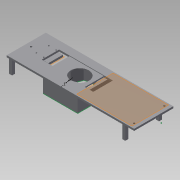
# Autodesk Inventor part: 10_Grundplatte
Saved by Autodesk Inventor 2015 (Build 190159000, 159)
## iProperties
Created: 2016-03-06
Part Number: 10_Grundplatte
Material: Generisch
Document SubType Name: Modeling
Designer: Bene
Density: 1 g/cm^3
Appearance: Vorgabe
Author: Bene
Autodesk Inventor part; units mm, degrees
ref_plane "YZ Plane" through (0, 0, 0) normal (1, 0, 0) x (0, 1, 0)
ref_plane "XZ Plane" through (0, 0, 0) normal (0, 1, 0) x (-1, 0, 0)
ref_plane "Arbeitsebene1" through (0, 0, 8) normal (0, 0, 1) x (1, 0, 0)
sketch "Skizze1" plane through (0, 0, 8) normal (0, 0, 1) x (1, 0, 0)
  arc A0 (2.5, 0) -> (0, 2.5) centre (0, 0) ccw projected
  line L0 (-80, 2.5) -> (0, 2.5) projected
  arc A1 (-80, 2.5) -> (-82.5, 0) centre (-80, 0) ccw projected
  line L1 (-82.5, -51) -> (-82.5, 0) projected
  arc A2 (-82.5, -51) -> (-80, -53.5) centre (-80, -51) ccw projected
  line L2 (0, -53.5) -> (-80, -53.5) projected
  arc A3 (0, -53.5) -> (2.5, -51) centre (0, -51) ccw projected
  line L3 (2.5, 0) -> (2.5, -51) projected
  circle A4 centre (-21, -1) radius 1.25 projected
  circle A5 centre (-79, -1) radius 1.25 projected
  circle A6 centre (-79, -50) radius 1.25 projected
  circle A7 centre (-21, -50) radius 1.25 projected
  line L4 (12.5, 7.5) -> (-177.5, 7.5)
  line L5 (-177.5, 7.5) -> (-177.5, -58.5)
  line L6 (-177.5, -58.5) -> (12.5, -58.5)
  line L7 (12.5, -58.5) -> (12.5, 7.5)
  dimension "d0" = 5
  dimension "d1" = 5
  dimension "d2" = 10
  dimension "d3" = 95
  constraints: 8 end point, 2 parallel, 1 horizontal, 1 perpendicular
  measures "d0" distance between parallel lines of L0 L4
  measures "d1" distance between parallel lines of L6 L2
  measures "d2" distance between parallel lines of L3 L7
  measures "d3" distance between parallel lines of L5 L1
extrude "Extrusion1" add sketch "Skizze1" against normal blind 3 contours L3 A3 L2 A2 L1 A1 L0 A0 | A4 | A5 | A6 | A7 | L7 L6 L5 L4
sketch "Skizze2" plane through (0, 0, 8) normal (0, 0, 1) x (1, 0, 0)
  line L0 (-112.1719, -23.0218) -> (-112.1719, -58.5) construction
  line L1 (12.5, -58.5) -> (-177.5, -58.5) construction
  line L2 (-112.1719, -23.0218) -> (-112.1719, 7.5) construction
  line L3 (-177.5, 7.5) -> (12.5, 7.5) construction
  circle A0 centre (-112.1719, -25.5) radius 12.8913 construction
  circle A1 centre (-112.1719, -25.5) radius 15.2609
  point P0 (0, 0)
  dimension "d6" = 66
  constraints: 4 end point, 4 point on line, 2 centre point, 1 coincident, 1 vertical
  measures "d6" distance between parallel lines of L3 L1
extrude "Extrusion2" cut sketch "Skizze2" against normal blind 3
sketch "Skizze3" plane through (0, 0, 5) normal (0, 0, -1) x (-1, 0, 0)
  circle A0 centre (79, -1) radius 1.25 projected
  circle A1 centre (79, -50) radius 1.25 projected
  circle A2 centre (21, -50) radius 1.25 projected
  circle A3 centre (21, -1) radius 1.25 projected
  circle A4 centre (79, -1) radius 3
  circle A5 centre (79, -50) radius 3
  circle A6 centre (21, -1) radius 3
  circle A7 centre (21, -50) radius 3
  point P0 (0, 0)
  dimension "d9" = 6
  dimension "d10" = 6
  dimension "d11" = 6
  dimension "d12" = 6
  constraints: 4 centre point, 4 coincident
  measures "d9" diameter of A4
  measures "d10" diameter of A5
  measures "d11" diameter of A6
  measures "d12" diameter of A7
ref_plane "Arbeitsebene2" through (-82.5, -53.5, 0) normal (0, 0, 1) x (1, 0, 0)
extrude "Extrusion3" add sketch "Skizze3" along normal up to surface (5 mm away) contours A0 | A1 | A2 | A3 | A4 | A5 | A6 | A7
sketch "Skizze4" plane through (-21, -50, 0) normal (0, 0, -1) x (-1, 0, 0)
  circle A0 centre (0, 49) radius 3 projected
  circle A1 centre (58, 49) radius 3 projected
  circle A2 centre (58, 0) radius 3 projected
  circle A3 centre (0, 0) radius 3 projected
  circle A4 centre (0, 49) radius 1
  circle A5 centre (58, 49) radius 1
  circle A6 centre (58, 0) radius 1
  circle A7 centre (0, 0) radius 1
  point P0 (-21, 50)
  dimension "d15" = 2
  dimension "d16" = 2
  dimension "d17" = 2
  dimension "d18" = 2
  constraints: 4 centre point
  measures "d15" radial gap between concentric circles of A0 A4
  measures "d16" radial gap between concentric circles of A1 A5
  measures "d17" radial gap between concentric circles of A2 A6
  measures "d18" radial gap between concentric circles of A3 A7
extrude "Extrusion4" add sketch "Skizze4" along normal blind 3 contours A4 | A5 | A6 | A7
sketch "Skizze8" plane through (0, 0, 5) normal (0, 0, -1) x (-1, 0, 0)
  line L0 (135.1719, -0.5) -> (93.1719, -0.5) construction
  line L1 (93.1719, -0.5) -> (93.1719, -50.5) construction
  line L2 (93.1719, -50.5) -> (135.1719, -50.5) construction
  line L3 (135.1719, -50.5) -> (135.1719, -0.5) construction
  line L4 (135.1719, -0.5) -> (93.1719, -50.5) construction
  line L5 (93.1719, -0.5) -> (135.1719, -50.5) construction
  circle A0 centre (135.1719, -0.5) radius 3.2
  circle A1 centre (135.1719, -50.5) radius 3.2
  circle A2 centre (93.1719, -0.5) radius 3.2
  circle A3 centre (93.1719, -50.5) radius 3.2
  circle A4 centre (112.1719, -25.5) radius 15 projected
  line L6 (144.3139, -20.5597) -> (134.048, -19.05)
  line L7 (134.048, -19.05) -> (128.1099, -2.846)
  line L8 (128.1099, -2.846) -> (116.7369, 0)
  line L9 (116.7369, 0) -> (96.3719, -7.4629)
  line L10 (96.3719, -7.4629) -> (92.1792, -14.1183)
  line L11 (92.1792, -14.1183) -> (87.8515, -27.8062)
  line L12 (87.8515, -27.8062) -> (96.3719, -47.0296)
  line L13 (96.3719, -47.0296) -> (110.7316, -51.5697)
  line L14 (110.7316, -51.5697) -> (144.3139, -44.1668)
  line L15 (144.3139, -44.1668) -> (144.3139, -20.5597)
  line L16 (143.0747, 5.5) -> (85.0747, 5.5)
  line L17 (85.0747, 5.5) -> (85.0747, -56.5)
  line L18 (85.0747, -56.5) -> (143.0747, -56.5)
  line L19 (143.0747, -56.5) -> (143.0747, 5.5)
  line L20 (143.0747, 5.5) -> (85.0747, -56.5) construction
  line L21 (85.0747, 5.5) -> (143.0747, -56.5) construction
  line L22 (200.5, -56.5) -> (195.5, -56.5)
  line L23 (195.5, -56.5) -> (195.5, -51.5)
  line L24 (195.5, -51.5) -> (200.5, -51.5)
  line L25 (200.5, -51.5) -> (200.5, -56.5)
  line L26 (177.5, -58.5) -> (177.5, 7.5) projected
  line L27 (200.5, 5.5) -> (195.5, 5.5)
  line L28 (195.5, 5.5) -> (195.5, 0.5)
  line L29 (195.5, 0.5) -> (200.5, 0.5)
  line L30 (200.5, 0.5) -> (200.5, 5.5)
  line L31 (4.5, 5.5) -> (9.5, 5.5)
  line L32 (9.5, 5.5) -> (9.5, 0.5)
  line L33 (9.5, 0.5) -> (4.5, 0.5)
  line L34 (4.5, 0.5) -> (4.5, 5.5)
  line L35 (4.5, -56.5) -> (9.5, -56.5)
  line L36 (9.5, -56.5) -> (9.5, -51.5)
  line L37 (9.5, -51.5) -> (4.5, -51.5)
  line L38 (4.5, -51.5) -> (4.5, -56.5)
  point P0 (0, 0)
  point P1 (114.1719, -25.5)
  point P2 (114.0747, -25.5)
  dimension "d24" = 42
  dimension "d25" = 50
  dimension "d26" = 6.4
  dimension "d27" = 6.4
  dimension "d28" = 6.4
  dimension "d29" = 6.4
  dimension "d30" = 2
  dimension "d31" = 0
  dimension "d32" = 58
  dimension "d33" = 62
  dimension "d34" = 0
  dimension "d44" = 5
  dimension "d46" = 5
  dimension "d47" = 5
  dimension "d48" = 5
  dimension "d49" = 5
  dimension "d50" = 5
  dimension "d51" = 5
  dimension "d52" = 5
  dimension "d56" = 0
  dimension "d57" = 23
  constraints: 76 end point, 12 parallel, 8 perpendicular, 6 horizontal, 4 centre point, 4 coincident, 3 midpoint, 2 point on line, 1 vertical
  measures "d24" distance of L2.end L1.end
  measures "d25" distance of L1.end L0.end
  measures "d26" diameter of A0
  measures "d27" diameter of A1
  measures "d28" diameter of A2
  measures "d29" diameter of A3
  measures "d30" distance of A4.centre point (114.172, -25.5)
  measures "d31" vertical distance of A4.centre point (114.172, -25.5)
  measures "d32" distance of L18.end L17.end
  measures "d33" distance of L17.end L16.end
  measures "d34" vertical distance of point (114.172, -25.5) point (114.075, -25.5)
  measures "d44" distance of L22.end L23.end
  measures "d46" distance between parallel lines of L25 L23
  measures "d47" distance of L29.end L28.end
  measures "d48" distance of L28.end L27.end
  measures "d49" distance of L32.end L33.end
  measures "d50" distance of L31.end L32.end
  measures "d51" distance of L37.end L36.end
  measures "d52" distance of L36.end L35.end
  measures "d56" distance between parallel lines of L30 L25
  measures "d57" distance between parallel lines of L25 L26
extrude "Extrusion6" add sketch "Skizze8" along normal blind 24 contours L6 L7 L8 L9 L10 L11 L12 L13 L14 L19 L18 L17 L16 | L22 L23 L24 L25 | L30 L29 L28 L27 | L31 L32 L33 L34 | L38 L37 L36 L35
sketch "Skizze9" plane through (0, 0, -19) normal (0, 0, -1) x (-1, 0, 0)
  line L0 (143.0747, -44.44) -> (110.7316, -51.5697) projected
  line L1 (110.7316, -51.5697) -> (96.3719, -47.0296) projected
  line L2 (96.3719, -47.0296) -> (87.8515, -27.8062) projected
  line L3 (87.8515, -27.8062) -> (92.1792, -14.1183) projected
  line L4 (92.1792, -14.1183) -> (96.3719, -7.4629) projected
  line L5 (96.3719, -7.4629) -> (116.7369, 0) projected
  line L6 (116.7369, 0) -> (128.1099, -2.846) projected
  line L7 (128.1099, -2.846) -> (134.048, -19.05) projected
  line L8 (134.048, -19.05) -> (143.0747, -20.3774) projected
  circle A0 centre (93.1719, -50.5) radius 3.2 projected
  circle A1 centre (93.1719, -0.5) radius 3.2 projected
  circle A2 centre (135.1719, -50.5) radius 3.2 projected
  circle A3 centre (135.1719, -0.5) radius 3.2 projected
  line L9 (143.0747, 5.5) -> (85.0747, 5.5) projected
  line L10 (85.0747, 5.5) -> (85.0747, -56.5) projected
  line L11 (85.0747, -56.5) -> (143.0747, -56.5) projected
  line L12 (143.0747, -20.3774) -> (143.0747, 5.5) projected
  line L13 (145.3139, -19.696) -> (145.3139, -44.9704)
  line L14 (145.3139, -44.9704) -> (110.6854, -52.6039)
  line L15 (110.6854, -52.6039) -> (95.6405, -47.8471)
  line L16 (95.6405, -47.8471) -> (86.7839, -27.8655)
  line L17 (86.7839, -27.8655) -> (91.2645, -13.6942)
  line L18 (91.2645, -13.6942) -> (95.7076, -6.6413)
  line L19 (95.7076, -6.6413) -> (116.6814, 1.0447)
  line L20 (116.6814, 1.0447) -> (128.8665, -2.0045)
  line L21 (128.8665, -2.0045) -> (134.7822, -18.1472)
  line L22 (134.7822, -18.1472) -> (145.3139, -19.696)
  line L23 (143.0747, -56.5) -> (143.0747, -44.44) projected
  point P0 (0, 0)
  dimension "d37" = 1
  constraints: 20 end point, 8 other
  measures "d37" distance between parallel lines of L8 L22
sketch "Skizze15" plane through (-177.5, -58.5, 8) normal (-1, 0, 0) x (0, 0, 1)
  line L0 (0, 66) -> (0, 0) projected
  line L1 (0, 66) -> (-3, 66) projected
  line L2 (-3, 0) -> (-3, 66) projected
  line L3 (0, 0) -> (-3, 0) projected
  point P0 (-8, 58.5)
extrude "Extrusion10" add sketch "Skizze15" along normal blind 25
ref_plane "Arbeitsebene3" through (-168.3757, -19.6, 1.6) normal (0, 0, 1) x (0, -1, 0)
sketch "Skizze16" plane through (-168.3757, -19.6, 1.6) normal (0, 0, 1) x (0, -1, 0)
  line L0 (-12.5, -14.5) -> (-12.5, 9.5) projected
  line L1 (-12.5, 9.5) -> (12.5, 9.5) projected
  line L2 (12.5, 9.5) -> (12.5, -14.5) projected
  line L3 (12.5, -14.5) -> (-12.5, -14.5) projected
  circle A0 centre (10.5, -12.5) radius 1.05 projected
  circle A1 centre (10.5, 0) radius 1.05 projected
  circle A2 centre (-10.5, 0) radius 1.05 projected
  circle A3 centre (-10.5, -12.5) radius 1.05 projected
  line L4 (8.7, -9.9) -> (7.48, -9.9) projected
  line L5 (8.7, -9.1) -> (8.7, -9.9) projected
  line L6 (7.48, -9.1) -> (8.7, -9.1) projected
  line L7 (7.48, -9.9) -> (7.48, -9.1) projected
  point P0 (-19.6, 168.3757)
  point P1 (-3.5315, -12.1603)
  constraints: 1 other
extrude "Extrusion11" add sketch "Skizze16" along normal up to surface (3.4 mm away)
sketch "Skizze17" plane through (0, 0, 5) normal (0, 0, -1) x (-1, 0, 0)
  circle A0 centre (168.3757, -9.1) radius 1.05 projected
  circle A1 centre (180.8757, -9.1) radius 1.05 projected
  circle A2 centre (180.8757, -30.1) radius 1.05 projected
  circle A3 centre (168.3757, -30.1) radius 1.05 projected
  line L0 (149.2615, -35.3027) -> (166.5964, -35.3027)
  line L1 (166.5964, -35.3027) -> (166.5964, -5.8969)
  line L2 (166.5964, -5.8969) -> (149.2615, -5.8969)
  line L3 (149.2615, -5.8969) -> (149.2615, -35.3027)
  line L4 (76.1083, -38.9253) -> (91.2151, -38.9253)
  line L5 (91.2151, -38.9253) -> (91.2151, -5.8969)
  line L6 (91.2151, -5.8969) -> (76.1083, -5.8969)
  line L7 (76.1083, -5.8969) -> (76.1083, -38.9253)
  point P0 (0, 0)
  constraints: 16 end point, 4 parallel, 2 horizontal, 2 perpendicular
extrude "Extrusion12" cut sketch "Skizze17" against normal blind 5
sketch "Skizze18" plane through (0, 0, 8) normal (0, 0, 1) x (1, 0, 0)
  line L0 (-91.2151, -38.9253) -> (-91.2151, -5.8969) projected
  line L1 (-91.2151, -5.8969) -> (-76.1083, -5.8969) projected
  line L2 (-76.1083, -5.8969) -> (-76.1083, -38.9253) projected
  line L3 (-76.1083, -38.9253) -> (-91.2151, -38.9253) projected
  circle A0 centre (-180.8757, -30.1) radius 1.05 projected
  circle A1 centre (-168.3757, -9.1) radius 1.05 projected
  circle A2 centre (-180.8757, -9.1) radius 1.05 projected
  circle A3 centre (-168.3757, -30.1) radius 1.05 projected
  line L4 (-166.5964, -35.3027) -> (-166.5964, -5.8969) projected
  line L5 (-166.5964, -5.8969) -> (-149.2615, -5.8969) projected
  line L6 (-149.2615, -5.8969) -> (-149.2615, -35.3027) projected
  line L7 (-149.2615, -35.3027) -> (-166.5964, -35.3027) projected
  circle A4 centre (-112.1719, -25.5) radius 15.2609 projected
  line L8 (12.5, 7.5) -> (-202.5, 7.5) projected
  line L9 (-202.5, -58.5) -> (-202.5, 7.5) projected
  line L10 (-202.5, -58.5) -> (12.5, -58.5) projected
  line L11 (12.5, -58.5) -> (12.5, 7.5) projected
  line L12 (-91.2151, -5.8969) -> (-149.2615, -5.8969)
  line L13 (-91.2151, -38.9253) -> (-149.2615, -35.3027)
  point P0 (0, 0)
  constraints: 4 end point, 1 horizontal
extrude "Extrusion13" cut sketch "Skizze18" against normal blind 1 contours L13 A4 L6 L12 L0 | L13 A4 picked at (-111.0612, -28.7224)
sketch "Skizze19" plane through (0, 0, 5) normal (0, 0, -1) x (-1, 0, 0)
  line L0 (122.2149, -36.9906) -> (149.2615, -35.3027) projected
  line L1 (149.2615, -35.3027) -> (166.5964, -35.3027) projected
  line L2 (166.5964, -35.3027) -> (166.5964, -5.8969) projected
  line L3 (166.5964, -5.8969) -> (76.1083, -5.8969) projected
  line L4 (76.1083, -5.8969) -> (76.1083, -38.9253) projected
  line L5 (76.1083, -38.9253) -> (91.2151, -38.9253) projected
  line L6 (91.2151, -38.9253) -> (103.6356, -38.1501) projected
  arc A0 (103.6356, -38.1501) -> (122.2149, -36.9906) centre (112.1719, -25.5) ccw projected
  circle A1 centre (180.8757, -30.1) radius 1.05 projected
  circle A2 centre (168.3757, -9.1) radius 1.05 projected
  circle A3 centre (180.8757, -9.1) radius 1.05 projected
  circle A4 centre (168.3757, -30.1) radius 1.05 projected
  line L7 (-12.5, 7.5) -> (202.5, 7.5) projected
  line L8 (202.5, -58.5) -> (202.5, 7.5) projected
  line L9 (202.5, -58.5) -> (-12.5, -58.5) projected
  line L10 (-12.5, -58.5) -> (-12.5, 7.5) projected
  circle A5 centre (-4.5, -50.5) radius 1.5
  circle A6 centre (-4.5, 0.5) radius 1.5
  circle A7 centre (194.5, -25.5) radius 1.5
  point P0 (0, 0)
  dimension "d64" = 3
  dimension "d65" = 3
  dimension "d66" = 3
  constraints: 3 centre point
  measures "d64" diameter of A5
  measures "d65" diameter of A6
  measures "d66" diameter of A7
extrude "Extrusion14" cut sketch "Skizze19" against normal through all contours A5 | A6 | A7
